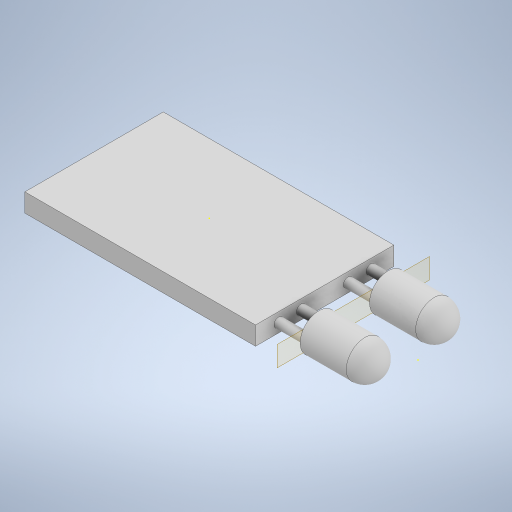
# Autodesk Inventor part: IR Sensor
Saved by Autodesk Inventor 2023 (Build 270158000, 158)
## iProperties
Created: 2022-06-16
Part Number: IR Sensor
Material: Generic
Document SubType Name: Modeling
Designer: chait
Density: 1 g/cm^3
Appearance: Default
Author: chait
Autodesk Inventor part; units mm, degrees
ref_plane "YZ Plane" through (0, 0, 0) normal (1, 0, 0) x (0, 1, 0)
ref_plane "XZ Plane" through (0, 0, 0) normal (0, 1, 0) x (-1, 0, 0)
ref_plane "XY Plane" through (0, 0, 0) normal (0, 0, 1) x (1, 0, 0)
sketch "Sketch1" plane through (0, 0, 0) normal (0, 1, 0) x (-1, 0, 0)
  line L0 (12.5, 7.5) -> (-12.5, 7.5)
  line L1 (-12.5, 7.5) -> (-12.5, -7.5)
  line L2 (-12.5, -7.5) -> (12.5, -7.5)
  line L3 (12.5, -7.5) -> (12.5, 7.5)
  line L4 (12.5, 7.5) -> (-12.5, -7.5) construction
  line L5 (-12.5, 7.5) -> (12.5, -7.5) construction
  point P0 (0, 0)
  dimension "d0" = 25
  dimension "d1" = 15
  constraints: 12 end point, 2 midpoint, 2 parallel, 1 horizontal, 1 perpendicular
  measures "d0" distance of L2.end L1.end
  measures "d1" distance of L1.end L0.end
extrude "Extrusion1" add sketch "Sketch1" along normal blind 2
sketch "Sketch2" plane through (12.5, 0, 7.5) normal (1, 0, 0) x (0, 0, -1)
  circle A0 centre (2.5013, 1) radius 0.5
  circle A1 centre (4.9343, 1) radius 0.5
  circle A2 centre (10.0214, 1) radius 0.5
  circle A3 centre (12.4987, 1) radius 0.5
  point P0 (7.5, 0)
  dimension "d4" = 1
  dimension "d5" = 1
  dimension "d6" = 1
  dimension "d7" = 1
  constraints: 4 centre point
  measures "d4" diameter of A0
  measures "d5" diameter of A1
  measures "d6" diameter of A2
  measures "d7" diameter of A3
extrude "Extrusion2" add sketch "Sketch2" along normal blind 3
ref_plane "Work Plane1" through (15.6, 0, 7.5) normal (1, 0, 0) x (0, 0, -1)
sketch "Sketch4" plane through (15.6, 0, 7.5) normal (1, 0, 0) x (0, 0, -1)
  circle A0 centre (3.7399, 1) radius 2
  circle A1 centre (11.2601, 1) radius 2
  point P0 (7.5, 0)
  dimension "d11" = 4
  dimension "d12" = 4
  constraints: 2 centre point
  measures "d11" diameter of A0
  measures "d12" diameter of A1
extrude "Extrusion3" add sketch "Sketch4" along normal blind 7
sketch "Sketch5" plane through (22.6, 1, 3.7601) normal (1, 0, 0) x (0, 0, -1)
  point P0 (3.7601, -1)
fillet "Fillet1" radius 2 1 edges at (22.6, 1, 5.7601)
fillet "Fillet2" radius 2 1 edges at (22.6, 1, -1.7601)
sketch "Sketch6" plane through (0, 2, 0) normal (0, 1, 0) x (1, 0, 0)
  point P0 (0, 0)
body "Solid1"
